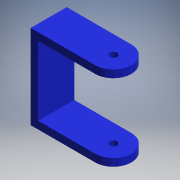
# Autodesk Inventor part: Middle_leg
Saved by Autodesk Inventor 2017 (Build 210142000, 142)
## iProperties
Part Number: Middle_leg
Material: Generic
Document SubType Name: Modeling
Designer: alex-
Appearance: Blue - Wall Paint - Glossy
Author: alex-
Autodesk Inventor part; units mm, degrees
ref_plane "YZ Plane" through (0, 0, 0) normal (1, 0, 0) x (0, 1, 0)
ref_plane "XZ Plane" through (0, 0, 0) normal (0, 1, 0) x (-1, 0, 0)
ref_plane "XY Plane" through (0, 0, 0) normal (0, 0, 1) x (1, 0, 0)
sketch "Sketch3" plane through (0, 0, 0) normal (0, 1, 0) x (-1, 0, 0)
  line L0 (2.5, 12) -> (-2.5, 12)
  line L1 (-2.5, 12) -> (-2.5, -12)
  line L2 (-2.5, -12) -> (2.5, -12)
  line L3 (2.5, -12) -> (2.5, 12)
  point P0 (0, 0)
  point P1 (0, 12)
  point P2 (2.5, 0)
  dimension "d6" = 5
  dimension "d7" = 24
  constraints: 8 end point, 2 midpoint, 2 parallel, 1 horizontal, 1 horizontal alignment, 1 perpendicular, 1 vertical alignment
  measures "d6" distance of L0.start L0.end
  measures "d7" distance of L2.end L0.start
extrude "Extrusion3" add sketch "Sketch3" along normal blind 56
sketch "Sketch4" plane through (2.5, 0, 12) normal (1, 0, 0) x (0, 0, -1)
  line L0 (0, 56) -> (24, 56)
  line L1 (24, 56) -> (24, 51)
  line L2 (24, 51) -> (0, 51)
  line L3 (0, 51) -> (0, 56)
  line L4 (0, 5) -> (24, 5)
  line L5 (24, 5) -> (24, 0)
  line L6 (24, 0) -> (0, 0)
  line L7 (0, 0) -> (0, 5)
  line L8 (0, 56) -> (24, 56) projected
  line L9 (0, 0) -> (24, 0) projected
  line L10 (0, 0) -> (0, 56) projected
  point P0 (12, 0)
  point P1 (12, 56)
  point P2 (12, 0)
  point P3 (12, 51)
  point P4 (12, 56)
  point P5 (12, 5)
  point P6 (12, 0)
  point P7 (0, 53.5)
  dimension "d10" = 5
  constraints: 16 end point, 9 midpoint, 4 parallel, 3 point on line, 2 horizontal, 2 perpendicular, 2 vertical alignment, 1 collinear
  measures "d10" distance of L0.end L1.end
extrude "Extrusion4" add sketch "Sketch4" along normal blind 50
fillet "Fillet1" radius 12 2 edges at (52.5, 53.5, 12) (52.5, 53.5, -12)
fillet "Fillet2" radius 12 2 edges at (52.5, 2.5, 12) (52.5, 2.5, -12)
sketch "Sketch6" plane through (0, 56, 0) normal (0, 1, 0) x (1, 0, 0)
  circle A0 centre (40.5, 0) radius 2.5
  arc A1 (40.5, -12) -> (40.5, 12) centre (40.5, 0) ccw projected
  point P0 (0, 0)
  dimension "d16" = 5
  constraints: 1 centre point, 1 concentric
  measures "d16" diameter of A0
extrude "Extrusion5" cut sketch "Sketch6" against normal up to surface (56 mm away) from surface at 0
equation "\"d6\" = b_mat_thickness"
equation "\"d7\" = sa_diameter"
equation "\"d8\" = sa_thickness + s_height + s_shaft_height + 2 * b_mat_thickness"
equation "\"d10\" = b_mat_thickness"
equation "\"d14\" = 0.5 * sa_diameter"
equation "\"d15\" = 0.5 * sa_diameter"
equation "\"b_mat_thickness\" = 5"
equation "\"sa_diameter\" = 24"
equation "\"sa_thickness\" = 2"
equation "\"s_height\" = 38"
equation "\"s_shaft_height\" = 6"
body "Solid2"
